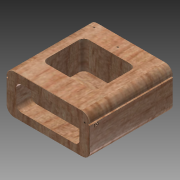
# Autodesk Inventor part: PassengerSectionDE
Saved by Autodesk Inventor 2015 (Build 190159000, 159)
## iProperties
Created: 2017-11-29
Part Number: PassengerSectionDE
Material: Generic
Document SubType Name: Modeling
Designer: Administrator
Density: 1 g/cm^3
Appearance: Default
Author: Administrator
Autodesk Inventor part; units mm, degrees
ref_plane "YZ Plane" through (0, 0, 0) normal (1, 0, 0) x (0, 1, 0)
ref_plane "XZ Plane" through (0, 0, 0) normal (0, 1, 0) x (-1, 0, 0)
ref_plane "XY Plane" through (0, 0, 0) normal (0, 0, 1) x (1, 0, 0)
sketch "Sketch1" plane through (0, 0, 0) normal (0, 0, 1) x (1, 0, 0)
  line L0 (7.62, 0) -> (72.898, 0)
  line L1 (80.518, 7.62) -> (80.518, 31.242)
  line L2 (72.898, 38.862) -> (7.62, 38.862)
  line L3 (0, 31.242) -> (0, 7.62)
  arc A0 (7.62, 38.862) -> (0, 31.242) centre (7.62, 31.242) ccw
  arc A1 (80.518, 31.242) -> (72.898, 38.862) centre (72.898, 31.242) ccw
  arc A2 (72.898, 0) -> (80.518, 7.62) centre (72.898, 7.62) ccw
  arc A3 (0, 7.62) -> (7.62, 0) centre (7.62, 7.62) ccw
  point P0 (0, 0)
  point P1 (80.518, 0)
  point P2 (0, 38.862)
  dimension "d0" = 38.862
  dimension "d1" = 80.518
  dimension "d2" = 7.62
  constraints: 8 end point, 8 point on circle, 8 tangent, 6 point on line, 4 centre point, 3 equal radius, 2 parallel, 1 horizontal, 1 perpendicular
  measures "d0" distance of point (0, 38.862) point (0, 0)
  measures "d1" distance of point (0, 0) point (80.518, 0)
  measures "d2" radius of A0
extrude "Extrusion1" add sketch "Sketch1" along normal blind 80.518
sketch "Sketch2" plane through (7.62, 38.862, 0) normal (0, 1, 0) x (1, 0, 0)
  line L0 (10.16, -58.7375) -> (50.292, -58.7375)
  line L1 (55.372, -53.6575) -> (55.372, -23.4315)
  line L2 (50.292, -18.3515) -> (10.16, -18.3515)
  line L3 (5.08, -23.4315) -> (5.08, -53.6575)
  arc A0 (5.08, -53.6575) -> (10.16, -58.7375) centre (10.16, -53.6575) ccw
  arc A1 (10.16, -18.3515) -> (5.08, -23.4315) centre (10.16, -23.4315) ccw
  arc A2 (55.372, -23.4315) -> (50.292, -18.3515) centre (50.292, -23.4315) ccw
  arc A3 (50.292, -58.7375) -> (55.372, -53.6575) centre (50.292, -53.6575) ccw
  point P0 (5.08, -58.7375)
  point P1 (55.372, -18.3515)
  point P2 (5.08, -18.3515)
  dimension "d7" = 50.292
  dimension "d8" = 40.386
  dimension "d10" = 5.08
  constraints: 8 end point, 8 point on circle, 8 tangent, 6 point on line, 4 centre point, 3 equal radius, 2 parallel, 1 horizontal, 1 perpendicular
  measures "d7" distance of point (55.372, -18.351) point (5.08, -18.352)
  measures "d8" distance of point (5.08, -18.352) point (5.08, -58.738)
  measures "d10" radius of A0
extrude "Extrusion2" cut sketch "Sketch2" against normal blind 27.178
sketch "Sketch3" plane through (0, 0, 80.518) normal (0, 0, 1) x (1, 0, 0)
  line L0 (14.732, 31.242) -> (65.532, 31.242)
  line L1 (70.612, 26.162) -> (70.612, 12.7)
  line L2 (65.532, 7.62) -> (14.732, 7.62)
  line L3 (9.652, 12.7) -> (9.652, 26.162)
  line L4 (0, 31.242) -> (0, 7.62) projected
  line L5 (7.62, 0) -> (72.898, 0) projected
  arc A0 (14.732, 31.242) -> (9.652, 26.162) centre (14.732, 26.162) ccw
  arc A1 (70.612, 26.162) -> (65.532, 31.242) centre (65.532, 26.162) ccw
  arc A2 (65.532, 7.62) -> (70.612, 12.7) centre (65.532, 12.7) ccw
  arc A3 (9.652, 12.7) -> (14.732, 7.62) centre (14.732, 12.7) ccw
  point P0 (0, 0)
  point P1 (9.652, 31.242)
  point P2 (70.612, 7.62)
  point P3 (9.652, 7.62)
  dimension "d17" = 23.622
  dimension "d18" = 60.96
  dimension "d19" = 9.652
  dimension "d20" = 7.62
  dimension "d21" = 5.08
  constraints: 8 end point, 8 point on circle, 8 tangent, 6 point on line, 4 centre point, 3 equal radius, 2 parallel, 1 horizontal, 1 perpendicular
  measures "d17" distance of point (9.652, 7.62) point (9.652, 31.242)
  measures "d18" distance of point (70.612, 7.62) point (9.652, 7.62)
  measures "d19" distance between parallel lines of L4 L3
  measures "d20" distance between parallel lines of L5 L2
  measures "d21" radius of A0
extrude "Extrusion3" cut sketch "Sketch3" against normal blind 14.478
sketch "Sketch4" plane through (0, 0, 0) normal (0, 0, -1) x (-1, 0, 0)
  line L0 (-67.056, 32.004) -> (-13.716, 32.004)
  line L1 (-8.636, 26.924) -> (-8.636, 11.684)
  line L2 (-13.716, 6.604) -> (-67.056, 6.604)
  line L3 (-72.136, 11.684) -> (-72.136, 26.924)
  line L4 (0, 7.62) -> (0, 31.242) projected
  line L5 (-72.898, 0) -> (-7.62, 0) projected
  arc A0 (-67.056, 32.004) -> (-72.136, 26.924) centre (-67.056, 26.924) ccw
  arc A1 (-8.636, 26.924) -> (-13.716, 32.004) centre (-13.716, 26.924) ccw
  arc A2 (-13.716, 6.604) -> (-8.636, 11.684) centre (-13.716, 11.684) ccw
  arc A3 (-72.136, 11.684) -> (-67.056, 6.604) centre (-67.056, 11.684) ccw
  point P0 (0, 0)
  point P1 (-8.636, 6.604)
  point P2 (-8.636, 32.004)
  point P3 (-72.136, 6.604)
  dimension "d24" = 63.5
  dimension "d25" = 25.4
  dimension "d26" = 8.636
  dimension "d27" = 6.604
  dimension "d28" = 5.08
  constraints: 8 end point, 8 point on circle, 8 tangent, 6 point on line, 4 centre point, 3 equal radius, 2 parallel, 1 horizontal, 1 perpendicular
  measures "d24" distance of point (-8.636, 6.604) point (-72.136, 6.604)
  measures "d25" distance of point (-8.636, 32.004) point (-8.636, 6.604)
  measures "d26" distance between parallel lines of L4 L1
  measures "d27" distance between parallel lines of L5 L2
  measures "d28" radius of A0
extrude "Extrusion4" cut sketch "Sketch4" against normal blind 14.478
sketch "Sketch5" plane through (80.518, 7.62, 0) normal (1, 0, 0) x (0, 0, -1)
  line L0 (-80.518, 23.622) -> (0, 23.622)
  line L1 (0, 23.622) -> (0, 22.098)
  line L2 (0, 22.098) -> (-80.518, 22.098)
  line L3 (-80.518, 22.098) -> (-80.518, 23.622)
  point P0 (0, -7.62)
  dimension "d31" = 1.524
  dimension "d32" = 80.518
  constraints: 8 end point, 2 parallel, 1 horizontal, 1 perpendicular
  measures "d31" distance of L0.end L1.end
  measures "d32" distance of L1.end L2.end
extrude "Extrusion5" cut sketch "Sketch5" against normal blind 1.524
sketch "Sketch6" plane through (0, 7.62, 0) normal (-1, 0, 0) x (0, 0, 1)
  line L0 (0, 23.622) -> (80.518, 23.622)
  line L1 (80.518, 23.622) -> (80.518, 22.098)
  line L2 (80.518, 22.098) -> (0, 22.098)
  line L3 (0, 22.098) -> (0, 23.622)
  point P0 (0, -7.62)
  dimension "d35" = 1.524
  dimension "d36" = 80.518
  constraints: 8 end point, 2 parallel, 1 horizontal, 1 perpendicular
  measures "d35" distance of L0.end L1.end
  measures "d36" distance of L1.end L2.end
extrude "Extrusion6" cut sketch "Sketch6" against normal blind 1.524
sketch "Sketch7" plane through (80.518, 7.62, 80.518) normal (1, 0, 0) x (0, 0, -1)
  line L0 (3.2137, 21.8083) -> (7.9488, 21.8083) construction
  line L1 (7.9488, 21.8083) -> (7.9488, 18.6393) construction
  line L2 (7.9488, 18.6393) -> (3.2137, 18.6393) construction
  line L3 (3.2137, 18.6393) -> (3.2137, 21.8083) construction
  line L4 (4.2338, 18.6986) -> (4.2338, 21.386)
  line L5 (4.2338, 21.386) -> (3.2113, 21.386)
  line L6 (3.2113, 21.386) -> (3.2113, 21.7466)
  line L7 (3.2113, 21.7466) -> (5.6615, 21.7466)
  line L8 (5.6615, 21.7466) -> (5.6615, 21.386)
  line L9 (5.6615, 21.386) -> (4.6389, 21.386)
  line L10 (4.6389, 21.386) -> (4.6389, 18.6986)
  line L11 (4.6389, 18.6986) -> (4.2338, 18.6986)
  spline S0 degree 2 poles (5.7998, 20.7561) (5.7998, 20.9908) (5.953, 21.381) (6.0864, 21.5218) knots 0 0 0 1 2 2 2
  spline S1 degree 2 poles (6.0864, 21.5218) (6.2123, 21.6577) (6.5804, 21.8083) (6.7681, 21.8083) knots 0 0 0 1 2 2 2
  spline S2 degree 2 poles (6.7681, 21.8083) (6.978, 21.8083) (7.3189, 21.6675) (7.4449, 21.5342) knots 0 0 0 1 2 2 2
  spline S3 degree 2 poles (7.4449, 21.5342) (7.603, 21.3662) (7.7759, 20.8228) (7.7759, 20.4054) knots 0 0 0 1 2 2 2
  spline S4 degree 2 poles (7.7759, 20.4054) (7.7759, 20.0274) (7.6054, 19.3507) (7.4399, 19.1259) knots 0 0 0 1 2 2 2
  spline S5 degree 2 poles (7.4399, 19.1259) (7.2646, 18.8888) (6.7706, 18.6393) (6.4099, 18.6393) knots 0 0 0 1 2 2 2
  spline S6 degree 2 poles (6.4099, 18.6393) (6.3284, 18.6393) (6.1432, 18.6566) (6.0641, 18.6813) knots 0 0 0 1 2 2 2
  line L12 (6.0641, 18.6813) -> (6.0641, 19.074)
  line L13 (6.0641, 19.074) -> (6.0839, 19.074)
  spline S7 degree 2 poles (6.0839, 19.074) (6.1358, 19.0444) (6.3531, 18.9925) (6.4643, 18.9925) knots 0 0 0 1 2 2 2
  spline S8 degree 2 poles (6.4643, 18.9925) (6.8644, 18.9925) (7.3214, 19.5211) (7.3535, 20.0102) knots 0 0 0 1 2 2 2
  spline S9 degree 2 poles (7.3535, 20.0102) (7.1905, 19.899) (6.8941, 19.7977) (6.7187, 19.7977) knots 0 0 0 1 2 2 2
  spline S10 degree 2 poles (6.7187, 19.7977) (6.5507, 19.7977) (6.2716, 19.8718) (6.1308, 19.978) knots 0 0 0 1 2 2 2
  spline S11 degree 2 poles (6.1308, 19.978) (5.9678, 20.104) (5.7998, 20.4869) (5.7998, 20.7561) knots 0 0 0 1 2 2 2
  spline S12 degree 2 poles (7.3634, 20.4968) (7.3634, 20.8055) (7.2497, 21.1958) (7.1485, 21.302) knots 0 0 0 1 2 2 2
  spline S13 degree 2 poles (7.1485, 21.302) (7.0595, 21.4008) (6.8743, 21.4749) (6.7656, 21.4749) knots 0 0 0 1 2 2 2
  spline S14 degree 2 poles (6.7656, 21.4749) (6.5137, 21.4749) (6.2148, 21.1143) (6.2148, 20.7734) knots 0 0 0 1 2 2 2
  spline S15 degree 2 poles (6.2148, 20.7734) (6.2148, 20.5807) (6.3136, 20.3313) (6.4223, 20.2423) knots 0 0 0 1 2 2 2
  spline S16 degree 2 poles (6.4223, 20.2423) (6.5013, 20.1781) (6.6965, 20.1361) (6.8101, 20.1361) knots 0 0 0 1 2 2 2
  spline S17 degree 2 poles (6.8101, 20.1361) (6.941, 20.1361) (7.2423, 20.2275) (7.3559, 20.3041) knots 0 0 0 1 2 2 2
  spline S18 degree 2 poles (7.3559, 20.3041) (7.3584, 20.3337) (7.3634, 20.435) (7.3634, 20.4968) knots 0 0 0 1 2 2 2
  point P0 (80.518, -7.62)
  constraints: 2 other
emboss "Emboss1" sketch "Sketch7" operation add depth 0.508 direction (-1, 0, 0)
chamfer "Chamfer1" distance 0.381 angle 45 3 edges at (40.259, 38.862, 80.518) (2.2318, 36.6302, 80.518) (78.2862, 36.6302, 80.518)
chamfer "Chamfer2" distance 0.381 angle 45 5 edges at (2.2318, 2.2318, 80.518) (40.259, 0, 80.518) (78.2862, 2.2318, 80.518) (80.518, 18.669, 80.518) (0, 18.669, 80.518)
chamfer "Chamfer3" distance 0.381 angle 45 3 edges at (40.259, 38.862, 0) (78.2862, 36.6302, 0) (2.2318, 36.6302, 0)
chamfer "Chamfer4" distance 0.381 angle 45 5 edges at (80.518, 18.669, 0) (78.2862, 2.2318, 0) (40.259, 0, 0) (2.2318, 2.2318, 0) (0, 18.669, 0)
body "Solid1"
